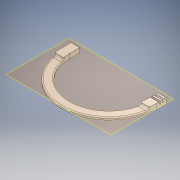
# Autodesk Inventor part: BottomCircleArmHalf
Saved by Autodesk Inventor 2017 (Build 210142000, 142)
## iProperties
Created: 2017-02-18
Part Number: BottomCircleArmHalf
Material: ABS Plastic
Document SubType Name: Modeling
Designer: aribu
Density: 1.06 g/cm^3
Appearance: Smooth - White
Author: aribu
Autodesk Inventor part; units mm, degrees
ref_plane "YZ Plane" through (0, 0, 0) normal (1, 0, 0) x (0, 1, 0)
ref_plane "XZ Plane" through (0, 0, 0) normal (0, 1, 0) x (-1, 0, 0)
ref_plane "XY Plane" through (0, 0, 0) normal (0, 0, 1) x (1, 0, 0)
sketch "Sketch1" plane through (0, 0, 0) normal (0, 0, 1) x (1, 0, 0)
  arc A0 (-41, 0) -> (41, 0) centre (0, 0) ccw
  arc A1 (-50, 0) -> (50, 0) centre (0, 0) ccw
  line L0 (-41, 0) -> (-41, 10)
  line L1 (41, 0) -> (41, 10)
  line L2 (-41, 10) -> (-50, 10)
  line L3 (-50, 10) -> (-50, 0)
  line L4 (-50, 0) -> (-50, 0)
  line L5 (41, 10) -> (50, 10)
  line L6 (50, 10) -> (50, 0)
  line L7 (50, 0) -> (50, 0)
  dimension "d0" = 82
  dimension "d1" = 100
  dimension "d12" = 9
  dimension "d13" = 9
  constraints: 16 end point, 4 perpendicular, 4 point on circle, 2 centre point, 2 coincident, 2 tangent, 1 horizontal, 1 vertical
  measures "d0" diameter of A0
  measures "d1" diameter of A1
  measures "d12" distance of L0.end L2.end
  measures "d13" distance of L1.end L5.end
extrude "Extrusion1" add sketch "Sketch1" along normal blind 12
sketch "Sketch2" plane through (50, 0, 0) normal (1, 0, 0) x (0, 0, -1)
  arc A0 (-3.5, -10) -> (-8.5, -10) centre (-6, -10) ccw
  line L0 (0, 10) -> (0, 0)
  line L1 (0, 0) -> (-10, 0)
  line L2 (-8.5, -10) -> (-8.5, -70)
  line L3 (-8.5, -70) -> (-3.5, -70)
  line L4 (-3.5, -70) -> (-3.5, -10)
  line L5 (0, 0) -> (-10, 0)
  line L6 (0, 10) -> (0, 0)
  dimension "d6" = 5
  dimension "d7" = 6
  dimension "d8" = 10
  dimension "d14" = 60
  dimension "d15" = 0
  dimension "d16" = 0
  dimension "d17" = 5
  constraints: 14 end point, 2 point on circle, 2 tangent, 1 centre point, 1 perpendicular, 1 vertical
  measures "d6" diameter of A0
  measures "d7" distance from line of L0 A0.centre
  measures "d8" distance from line of L1 A0.centre
  measures "d14" distance of L2.start L2.end
  measures "d15" distance between parallel lines of L5 L1
  measures "d16" distance between parallel lines of L6 L0
  measures "d17" distance of L2.end L3.end
extrude "Extrusion2" cut sketch "Sketch2" against normal blind 100
fillet "Fillet1" radius 1 16 edges at (40.3082, -7.5, 5.9921) (0, -41, 8.5) (-40.3082, -7.5, 5.9921) (0, -41, 3.5) (-49.4343, -7.5, 6) (0, -50, 8.5) (49.4343, -7.5, 6) (0, -50, 3.5) (0, -50, 12) (0, -50, 0) (41, 5, 0) (-41, 5, 0) (0, -41, 0) (-41, 5, 12) (41, 5, 12) (0, -41, 12)
sketch "Sketch3" plane through (50, 0, 1) normal (1, 0, 0) x (0, 0, -1)
  line L0 (-11, 10) -> (-11, 0) projected
  line L1 (0, 10) -> (-10, 10) projected
  line L2 (-7.7753, 4) -> (-2.2247, 4)
  line L3 (-2.2247, 6) -> (-7.7753, 6)
  arc A0 (-7.7753, 4) -> (-2.2247, 4) centre (-5, 5) ccw
  arc A1 (-2.2247, 6) -> (-7.7753, 6) centre (-5, 5) ccw
  point P0 (1, 0)
  dimension "d18" = 6
  dimension "d19" = 5
  constraints: 4 end point, 4 point on circle, 2 centre point, 1 horizontal, 1 parallel
  measures "d18" distance from line of L0 A0.centre
  measures "d19" distance from line of L1 A0.centre
extrude "Extrusion3" cut sketch "Sketch3" against normal blind 10
ref_plane "Work Plane1" through (0, 0, 6) normal (0, 0, 1) x (1, 0, 0)
split "Split1" plane through (0, 0, 6) removes the side toward (0, 0, 1)
body "Solid1"
